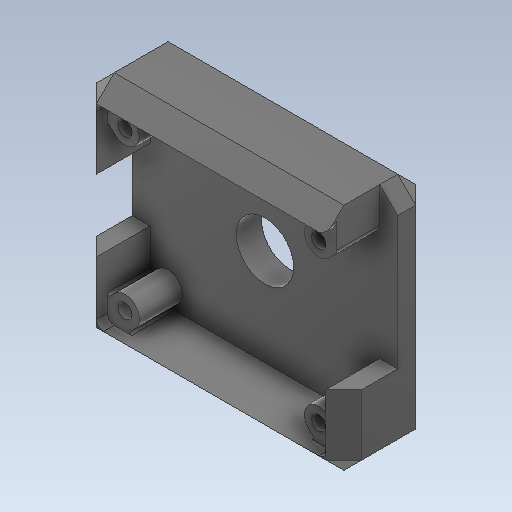
# Autodesk Inventor part: Camera_cover_01
Saved by Autodesk Inventor 2020.4 (Build 244396000, 396)
## iProperties
Created: 2021-08-25
Part Number: Camera_cover_01
Material: アセタール樹脂、黒
Document SubType Name: Modeling
Designer: t-nagamine
Density: 1.425 g/cm^3
Appearance: 滑らか - 黒
Description: PLA
Author: t-nagamine
Autodesk Inventor part; units mm, degrees
ref_plane "YZ Plane" through (0, 0, 0) normal (1, 0, 0) x (0, 1, 0)
ref_plane "XZ Plane" through (0, 0, 0) normal (0, 1, 0) x (-1, 0, 0)
ref_plane "XY Plane" through (0, 0, 0) normal (0, 0, 1) x (1, 0, 0)
sketch "スケッチ1" plane through (0, 0, 0) normal (0, 0, 1) x (1, 0, 0)
  line L0 (-37, 32) -> (37, 32)
  line L1 (37, 32) -> (37, -32)
  line L2 (37, -32) -> (-37, -32)
  line L3 (-37, -32) -> (-37, 32)
  line L4 (-37, 32) -> (37, -32) construction
  line L5 (37, 32) -> (-37, -32) construction
  line L6 (-32, 27) -> (32, 27)
  line L7 (32, 27) -> (32, -27)
  line L8 (32, -27) -> (-32, -27)
  line L9 (-32, -27) -> (-32, 27)
  line L10 (-32, 27) -> (32, -27) construction
  line L11 (32, 27) -> (-32, -27) construction
  arc A0 (-30, 27) -> (-32, 25) centre (-30, 25) ccw
  line L12 (0, 32) -> (0, -32) construction
  line L13 (37, 0) -> (-37, 0) construction
  arc A1 (-32, -25) -> (-30, -27) centre (-30, -25) ccw
  arc A2 (32, 25) -> (30, 27) centre (30, 25) ccw
  arc A3 (30, -27) -> (32, -25) centre (30, -25) ccw
  circle A4 centre (-27, 22) radius 2
  circle A5 centre (-27, 22) radius 4
  line L14 (-32, 21.3431) -> (-29.8284, 19.1716)
  line L15 (-26.3431, 27) -> (-24.1716, 24.8284)
  circle A6 centre (-27, -22) radius 2
  circle A7 centre (-27, -22) radius 4
  line L16 (-32, -21.3431) -> (-29.8284, -19.1716)
  line L17 (-26.3431, -27) -> (-24.1716, -24.8284)
  line L18 (32, 27) -> (-32, -27) construction
  circle A8 centre (27, 22) radius 2
  circle A9 centre (27, 22) radius 4
  line L19 (32, 21.3431) -> (29.8284, 19.1716)
  line L20 (26.3431, 27) -> (24.1716, 24.8284)
  circle A10 centre (27, -22) radius 4
  circle A11 centre (27, -22) radius 2
  line L21 (26.3431, -27) -> (24.1716, -24.8284)
  line L22 (32, -21.3431) -> (29.8284, -19.1716)
  circle A12 centre (0, 0) radius 8
  line L23 (-32, 10) -> (-37, 10)
  line L24 (-32, -10) -> (-37, -10)
  line L25 (24, 15) -> (-24, 15)
  line L26 (-24, 15) -> (-24, -15)
  line L27 (-24, -15) -> (24, -15)
  line L28 (24, -15) -> (24, 15)
  line L29 (24, 15) -> (-24, -15) construction
  line L30 (-24, 15) -> (24, -15) construction
  line L31 (24, 10) -> (19, 15)
  line L32 (24, -10) -> (19, -15)
  line L33 (-24, 10) -> (-19, 15)
  line L34 (-24, -10) -> (-19, -15)
  line L35 (32, -10) -> (37, -10)
  line L36 (32, 27) -> (32, 32)
  dimension "d1" = 64
  dimension "d3" = 54
  dimension "d4" = 74
  dimension "d5" = 64
  dimension "d6" = 2
  dimension "d7" = 2
  dimension "d8" = 2
  dimension "d9" = 10
  dimension "d10" = 10
  dimension "d11" = 4
  dimension "d12" = 8
  dimension "d13" = 45
  dimension "d14" = 45
  dimension "d15" = 16
  dimension "d17" = 20
  dimension "d31" = 48
  dimension "d32" = 30
  dimension "d40" = 5
  dimension "d41" = 5
  constraints: 74 end point, 37 symmetric about line, 16 point on circle, 13 centre point, 10 midpoint, 10 point on line, 6 coincident, 6 parallel, 4 perpendicular, 3 horizontal, 2 tangent, 9 other
  measures "d1" distance of L2.end L0.start
  measures "d3" distance of L8.end L6.start
  measures "d4" distance of L1.end L2.end
  measures "d5" distance of L7.end L8.end
  measures "d6" radius of A0
  measures "d7" distance of L6.start A0.start
  measures "d8" distance of A0.end L6.start
  measures "d9" distance from line of L0 point (-27, 22)
  measures "d10" distance from line of L3 point (-27, 22)
  measures "d11" diameter of A4
  measures "d12" diameter of A5
  measures "d13" angle of L9 L14
  measures "d14" angle of L6 L15
  measures "d15" diameter of A12
  measures "d17" distance between parallel lines of L23 L24
  measures "d31" distance of L27.end L26.end
  measures "d32" distance of L27.end L25.start
  measures "d40" distance of L25.start L31.end
  measures "d41" distance of L25.start L31.start
extrude "押し出し2" add sketch "スケッチ1" along normal blind 15 contours L0 L36 L6 L9 L23 L3 | L24 L9 L8 L7 L35 L1 L2 L3 | L9 L6 A0 | A1 L8 L9 | L7 L8 A3
extrude "押し出し3" add sketch "スケッチ1" along normal blind 12 contours L7 A2 L6 | A2 L7 L19 A9 L20 L6 | L9 A0 L6 L15 A5 L14 | L16 A7 L17 L8 A1 L9 | L9 L6 A0 | A5 | L7 A3 L8 L21 A10 L22 | A9 | A1 L8 L9 | A7 | A10
extrude "押し出し7" add sketch "スケッチ1" against normal blind 10 contours L0 L36 L6 L9 L23 L3 | L0 L1 L35 L7 L36 | L23 L9 L24 L3 | L7 A2 L6 | L24 L9 L8 L7 L35 L1 L2 L3 | L9 L14 A5 L15 L6 L20 A9 L19 L7 L22 A10 L21 L8 L17 A7 L16 | A2 L7 L19 A9 L20 L6 | L9 A0 L6 L15 A5 L14 | L16 A7 L17 L8 A1 L9 | L9 L6 A0 | A5 | L7 A3 L8 L21 A10 L22 | A9 | A1 L8 L9 | A7 | L7 L8 A3 | A10 | A4 | A6 | A8 | A11 | L28 L31 L25 | L33 L26 L25 | L28 L27 L32 | L34 L27 L26
extrude "押し出し9" add sketch "スケッチ1" against normal blind 7 contours L31 L28 L32 L27 L34 L26 L33 L25
chamfer "面取り1" distance 5 angle 45 13 edges at (0, -32, 15) (37, -21, 15) (-2.5, 32, 15) (-37, -21, 15) (-37, 21, 15) (-37, 32, 2.5) (-37, -32, 2.5) (37, -32, 2.5) (37, 32, -5) (37, 0, -10) (0, -32, -10) (-37, 0, -10) (0, 32, -10)
fillet "フィレット2" radius 0.5 7 edges at (-26.3431, -27, 6) (-32, -21.3431, 6) (-32, 21.3431, 6) (-26.3431, 27, 6) (26.3431, 27, 6) (26.3431, -27, 6) (32, -21.3431, 6)
fillet "フィレット3" radius 2 8 edges at (-19, 15, -8.5) (-24, 10, -8.5) (-24, -10, -8.5) (-19, -15, -8.5) (19, -15, -8.5) (24, -10, -8.5) (24, 10, -8.5) (19, 15, -8.5)
fillet "フィレット4" radius 2 2 edges at (32, 27, 13.5) (32, 21.3431, 6)
equation "\"d10\" = d9"
